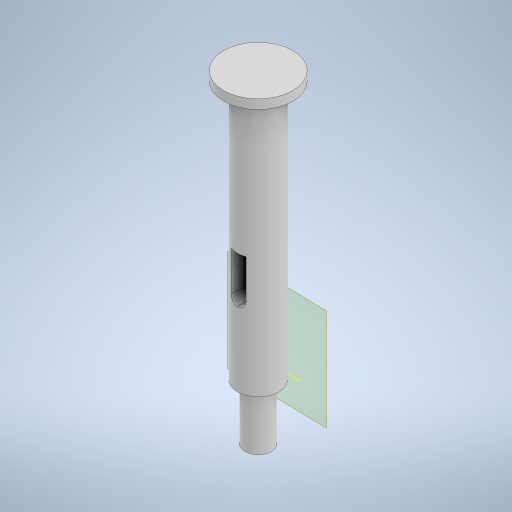
# Autodesk Inventor part: pin
Saved by Autodesk Inventor 2023 (Build 270158000, 158)
## iProperties
Created: 2025-10-02
Part Number: pin
Material: Generic
Document SubType Name: Modeling
Designer: ptato_qo49uko
Density: 1 g/cm^3
Appearance: Default
Author: ptato_qo49uko
Autodesk Inventor part; units mm, degrees
ref_plane "YZ Plane" through (0, 0, 0) normal (1, 0, 0) x (0, 1, 0)
ref_plane "XZ Plane" through (0, 0, 0) normal (0, 1, 0) x (-1, 0, 0)
ref_plane "XY Plane" through (0, 0, 0) normal (0, 0, 1) x (1, 0, 0)
sketch "Sketch1" plane through (0, 0, 0) normal (0, 1, 0) x (-1, 0, 0)
  circle A0 centre (0, 0) radius 7.5
  dimension "d0" = 15
  constraints: 1 centre point, 1 coincident
  measures "d0" diameter of A0
extrude "Extrusion1" add sketch "Sketch1" along normal blind 2
sketch "Sketch2" plane through (0, 0, 0) normal (0, -1, 0) x (1, 0, 0)
  circle A0 centre (0, 0) radius 4.5
  constraints: 1 centre point, 1 coincident
extrude "Extrusion2" add sketch "Sketch2" along normal blind 68
sketch "Sketch4" plane through (0, 2, 0) normal (0, 1, 0) x (1, 0, 0)
  circle A0 centre (0, 0) radius 4.5
  circle A1 centre (0, 0) radius 4.5 projected
  line L0 (-1.6, -4.2059) -> (-1.6, 4.2059)
  line L1 (1.6, -4.2059) -> (1.6, 4.2059)
  dimension "d6" = 9
  constraints: 4 end point, 4 point on circle, 2 vertical, 1 centre point, 1 coincident
  measures "d6" diameter of A0
extrude "Extrusion3" cut sketch "Sketch4" against normal blind 42 contours L1 A0 L0
sketch "Sketch5" plane through (0, 2, 0) normal (0, 1, 0) x (1, 0, 0)
  circle A0 centre (0, 0) radius 4.5
  arc A1 (-1.6, -4.2059) -> (1.6, -4.2059) centre (0, 0) ccw projected
  line L0 (-1.6, -4.2059) -> (-1.6, 4.2059) projected
  line L1 (-1.6, -4.2059) -> (-1.6, 4.2059)
  line L2 (1.6, 4.2059) -> (1.6, -4.2059) projected
  arc A2 (1.6, 4.2059) -> (-1.6, 4.2059) centre (0, 0) ccw projected
  line L3 (1.6, -4.2059) -> (1.6, 4.2059)
  dimension "d9" = 9
  constraints: 4 end point, 1 centre point, 1 coincident, 1 collinear
  measures "d9" diameter of A0
extrude "Extrusion4" add sketch "Sketch5" against normal blind 32 contours L2 A0 L0
fillet "Fillet1" radius 1.5 1 edges at (-1.6, -40, 0)
fillet "Fillet2" radius 1.499 1 edges at (1.6, -40, 0)
sketch "Sketch6" plane through (0, -40, 0) normal (0, 1, 0) x (1, 0, 0)
  point P0 (0, 0)
ref_plane "Work Plane2" through (0.101, -40, -4.4989) normal (0.0224, 0, -0.9997) x (0, 1, 0)
sketch "Sketch8" plane through (0, -68, 0) normal (0, -1, 0) x (1, 0, 0)
  circle A0 centre (0, 0) radius 2.875
  circle A1 centre (0, 0) radius 4.5
  dimension "d23" = 5.75
  constraints: 2 centre point, 2 coincident
  measures "d23" diameter of A0
extrude "Extrusion5" cut sketch "Sketch8" against normal blind 12
sketch "Sketch9" plane through (0.101, -40, -4.4989) normal (0.0224, 0, -0.9997) x (0, 1, 0)
  line L0 (-16, -4.5) -> (-16, 4.5) projected
  line L1 (-16, 0) -> (10, -0.0944)
  line L2 (10, 1.5052) -> (10, -1.694) projected
  point P0 (40, 0)
  constraints: 2 end point, 2 midpoint
body "Solid1"
